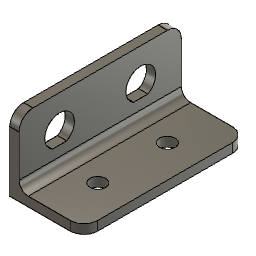
BaseAntennaMount (Autodesk Fusion 360 design; units mm, degrees)
Autodesk Fusion 360 part; units mm, degrees
note: some values were not read from the file. Set by a fixed rule: which sketch regions a step uses.
sketch "Sketch1" plane through (0, 0, 0) normal (0, 0, 1) x (1, 0, 0)
  line L0 (0, 0) -> (16, 0)
  line L1 (16, 0) -> (16, 2)
  line L2 (16, 2) -> (2, 2)
  line L3 (2, 2) -> (2, 16)
  line L4 (2, 16) -> (0, 16)
  line L5 (0, 16) -> (0, 0)
  dimension "d1" = 16
  dimension "d2" = 16
  dimension "d3" = 2
  dimension "d4" = 2
  constraint coincident L0.start L5.end
  constraint horizontal L0
  constraint perpendicular L0 L1
  constraint perpendicular L1 L2
  constraint perpendicular L2 L3
  constraint perpendicular L3 L4
  constraint perpendicular L0 L5
  measures "d1" distance of L4.end L0.start
  measures "d2" distance of L0.start L0.end
  measures "d3" distance of L0.end L1.end
  measures "d4" distance of L3.end L4.end
extrude "Extrude1" add sketch "Sketch1" against normal blind 35
sketch "Sketch2" plane through (0, 2, 0) normal (0, 1, 0) x (-1, 0, 0)
  line L0 (-2, 0) -> (-16, 0)
  line L1 (-16, 0) -> (-16, -35)
  line L2 (-16, -35) -> (-2, -35)
  line L3 (-2, -35) -> (-2, 0)
  line L4 (-9, -35) -> (-9, 0) construction
  line L5 (-16, -17.5) -> (-2, -17.5) construction
  circle A0 centre (-9, -10) radius 1.7
  circle A1 centre (-9, -25) radius 1.7
  dimension "d7" = 3.4
  dimension "d19" = 7.5
  constraint midpoint L2 L4.start
  constraint midpoint L0 L4.end
  constraint midpoint L1 L5.start
  constraint midpoint L3 L5.end
  constraint coincident L4 A0.centre
  constraint symmetric L5 A0 A1
  measures "d7" diameter of A0
  measures "d19" distance of L5 A0.centre
extrude "Extrude2" cut sketch "Sketch2" against normal blind 2 contours A0 | A1
sketch "Sketch3" plane through (2, 0, 0) normal (1, 0, 0) x (0, 0, -1)
  line L0 (0, 16) -> (0, 2)
  line L1 (0, 2) -> (35, 2)
  line L2 (35, 2) -> (35, 16)
  line L3 (35, 16) -> (0, 16)
  line L4 (17.5, 16) -> (17.5, 2) construction
  line L5 (0, 9) -> (35, 9) construction
  circle A0 centre (8.75, 9) radius 3.2
  line L6 (0, 12.2) -> (35, 12.2) construction
  line L7 (0, 6.2) -> (35, 6.2) construction
  line L8 (7.2008, 6.2) -> (10.2992, 6.2)
  circle A1 centre (26.25, 9) radius 3.2
  line L9 (27.7992, 6.2) -> (24.7008, 6.2)
  dimension "d10" = 6.4
  dimension "d11" = 6
  dimension "d12" = 8.75
  constraint midpoint L3 L4.start
  constraint midpoint L1 L4.end
  constraint midpoint L0 L5.start
  constraint midpoint L2 L5.end
  constraint coincident L5 A0.centre
  constraint coincident L0 L6.start
  constraint coincident L2 L6.end
  constraint perpendicular L2 L6
  constraint coincident L0 L7.start
  constraint coincident L2 L7.end
  constraint perpendicular L2 L7
  constraint tangent A0 L6
  constraint coincident L7 L8.start
  constraint coincident A0 L8.start
  constraint coincident L7 L8.end
  constraint coincident A0 L8.end
  constraint symmetric L4 A0 A1
  constraint symmetric L4 L8.start L9.start
  constraint symmetric L4 L8.end L9.end
  measures "d10" diameter of A0
  measures "d11" distance of L6 L7
  measures "d12" distance of L4 A0.centre
extrude "Extrude3" cut sketch "Sketch3" against normal blind 2 contours A0 L8 | A1 L9 picked at (8.5695, 8.1846) picked at (27.2186, 9.3965)
fillet "Fillet1" radius 2 1 edges at (2, 2, -17.5)
fillet "Fillet2" radius 3 4 edges at (1, 16, -35) (1, 16, 0) (16, 1, 0) (16, 1, -35)
equation "d12 = ( 17.5 / 2 ) * 1 mm"
equation "d19 = ( 15 / 2 ) * 1 mm"
